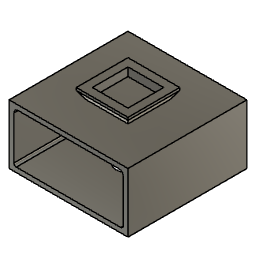
Base_station_adapter v7 (Autodesk Fusion 360 design; units mm, degrees)
Autodesk Fusion 360 part; units mm, degrees
sketch "Sketch1" plane through (0, 0, 0) normal (0, 0, 1) x (1, 0, 0)
  line L0 (-50, -50) -> (50, -50)
  line L1 (50, -50) -> (50, 50)
  line L2 (50, 50) -> (-50, 50)
  line L3 (-50, 50) -> (-50, -50)
  dimension "d1" = 100
  dimension "d2" = 100
  dimension "d3" = 50
  dimension "d4" = 50
  constraint horizontal L0
  constraint vertical L1
  constraint horizontal L2
  constraint vertical L3
  measures "d1" distance of L1.end L2.end
  measures "d2" distance of L0.start L2.end
  measures "d3" distance of origin L1
  measures "d4" distance of origin L0
extrude "Extrude1" add sketch "Sketch1" along normal blind 50
sketch "Sketch2" plane through (0, -50, 0) normal (0, -1, 0) x (1, 0, 0)
  line L0 (-50, 0) -> (50, 0)
  line L1 (50, 0) -> (50, 50)
  line L2 (50, 50) -> (-50, 50)
  line L3 (-50, 50) -> (-50, 0)
  line L4 (-46, 46) -> (46, 46)
  line L5 (46, 46) -> (46, 4)
  line L6 (46, 4) -> (-46, 4)
  line L7 (-46, 4) -> (-46, 46)
  dimension "d7" = 92
  dimension "d8" = 46
  dimension "d10" = 4
  dimension "d58" = 4
  constraint horizontal L4
  constraint vertical L5
  constraint horizontal L6
  constraint vertical L7
  measures "d7" distance of L4.start L4.end
  measures "d8" distance of origin L7
  measures "d10" distance of L2 L4
  measures "d58" distance of L0 L6
extrude "Extrude2" cut sketch "Sketch2" against normal blind 96 contours L4 L5 L6 L7
sketch "Sketch4" plane through (0, 0, 50) normal (0, 0, 1) x (-1, 0, 0)
  line L0 (50, -50) -> (50, 50)
  line L1 (50, 50) -> (-50, 50)
  line L2 (-50, 50) -> (-50, -50)
  line L3 (-50, -50) -> (50, -50)
  circle A0 centre (0, 0) radius 6
  dimension "d23" = 12
  constraint coincident A0.centre origin
  measures "d23" diameter of A0
hole "Hole1" at (0, 0, 50) direction (0, 0, -1) diameter 20 depth 4 tip angle 118
fillet "Fillet2" radius 3.5 3 edges at (0, 46, 4) (-46, -2, 4) (46, -2, 4)
fillet "Fillet4" radius 2 3 edges at (-46, -2, 46) (0, 46, 46) (46, -2, 46)
sketch "Sketch10" plane through (0, 0, 0) normal (0, 0, -1) x (1, 0, 0)
  line L0 (-50, 50) -> (-50, -50)
  line L1 (-50, -50) -> (50, -50)
  line L2 (50, -50) -> (50, 50)
  line L3 (50, 50) -> (-50, 50)
  line L4 (-17.5, 17.5) -> (17.5, 17.5)
  line L5 (17.5, 17.5) -> (17.5, -17.5)
  line L6 (17.5, -17.5) -> (-17.5, -17.5)
  line L7 (-17.5, -17.5) -> (-17.5, 17.5)
  dimension "d105" = 35
  dimension "d106" = 35
  dimension "d107" = 17.5
  dimension "d108" = 17.5
  constraint horizontal L4
  constraint vertical L5
  constraint horizontal L6
  constraint vertical L7
  measures "d105" distance of L4.start L4.end
  measures "d106" distance of L4.end L5.end
  measures "d107" distance of origin L4
  measures "d108" distance of origin L5
extrude "Extrude8" add sketch "Sketch10" along normal blind 9 draft 32 contours L4 L5 L6 L7
sketch "Sketch12" plane through (0, 0, -9) normal (0, 0, -1) x (1, 0, 0)
  line L0 (-23.1238, 23.1238) -> (-23.1238, -23.1238)
  line L1 (-23.1238, -23.1238) -> (23.1238, -23.1238)
  line L2 (23.1238, -23.1238) -> (23.1238, 23.1238)
  line L3 (23.1238, 23.1238) -> (-23.1238, 23.1238)
  line L4 (-21.75, 21.75) -> (21.75, 21.75)
  line L5 (21.75, 21.75) -> (21.75, -21.75)
  line L6 (21.75, -21.75) -> (-21.75, -21.75)
  line L7 (-21.75, -21.75) -> (-21.75, 21.75)
  dimension "d111" = 43.5
  dimension "d112" = 43.5
  dimension "d113" = 21.75
  dimension "d114" = 21.75
  constraint horizontal L4
  constraint vertical L5
  constraint horizontal L6
  constraint vertical L7
  measures "d111" distance of L4.start L4.end
  measures "d112" distance of L4.end L5.end
  measures "d113" distance of origin L5
  measures "d114" distance of origin L4
extrude "Extrude9" cut sketch "Sketch12" against normal blind 9
move_body "Move2" bodies 1 to x (-1, 0, 0) y (0, 1, 0) z (0, 0, -1) at (0, 0, 4)
sketch "Sketch15" plane through (0, 0, 13) normal (0, 0, 1) x (-1, 0, 0)
  line L0 (-21.75, 21.75) -> (-21.75, -21.75)
  line L1 (-21.75, -21.75) -> (21.75, -21.75)
  line L2 (21.75, -21.75) -> (21.75, 21.75)
  line L3 (21.75, 21.75) -> (-21.75, 21.75)
  line L4 (15, -15) -> (-15, -15)
  line L5 (-15, -15) -> (-15, 15)
  line L6 (-15, 15) -> (15, 15)
  line L7 (15, 15) -> (15, -15)
  constraint horizontal L4
  constraint vertical L5
  constraint horizontal L6
  constraint vertical L7
extrude "Extrude12" cut sketch "Sketch15" against normal blind 7 contours L4 L5 L6 L7
